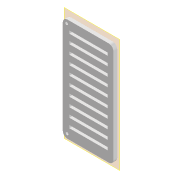
# Autodesk Inventor part: 00_Case_Powersupply_Galvo_lid
Saved by Autodesk Inventor 2022 (Build 260153000, 153)
## iProperties
Created: 2021-10-08
Part Number: 00_Case_Powersupply_Galvo_lid
Material: Generic
Document SubType Name: Modeling
Designer: wanghaoran
Density: 1 g/cm^3
Appearance: Default
Author: wanghaoran
Autodesk Inventor part; units mm, degrees
ref_plane "YZ Plane" through (0, 0, 0) normal (1, 0, 0) x (0, 1, 0)
ref_plane "XZ Plane" through (0, 0, 0) normal (0, 1, 0) x (-1, 0, 0)
ref_plane "XY Plane" through (0, 0, 0) normal (0, 0, 1) x (1, 0, 0)
ref_plane "Work Plane1" through (0, 0, 0) normal (0, 0, 1) x (1, 0, 0)
sketch "Sketch1" plane through (0, 0, 0) normal (0, 0, 1) x (1, 0, 0)
  circle A0 centre (-23, 51) radius 1.45 projected
  circle A1 centre (-22.4561, -50.4561) radius 1.45 projected
  arc A2 (-27, -50) -> (-22, -55) centre (-22, -50) ccw projected
  line L0 (-22, -55) -> (22, -55) projected
  arc A3 (22, -55) -> (27, -50) centre (22, -50) ccw projected
  line L1 (27, -50) -> (27, 50) projected
  arc A4 (27, 50) -> (22, 55) centre (22, 50) ccw projected
  line L2 (22, 55) -> (-22, 55) projected
  arc A5 (-22, 55) -> (-27, 50) centre (-22, 50) ccw projected
  line L3 (-27, 50) -> (-27, -50) projected
  line L4 (-22, 53) -> (22, 53) projected
  arc A6 (25, 50) -> (22, 53) centre (22, 50) ccw projected
  line L5 (25, 50) -> (25, -50) projected
  arc A7 (22, -53) -> (25, -50) centre (22, -50) ccw projected
  line L6 (22, -53) -> (-22, -53) projected
  arc A8 (-22, -53) -> (-25, -50) centre (-22.4561, -50.4561) ccw projected
  line L7 (-25, -50) -> (-25, 50) projected
  arc A9 (-25, 50) -> (-22, 53) centre (-23, 51) ccw projected
  point P0 (0, 0)
extrude "Extrusion1" add sketch "Sketch1" along normal blind 4 contours L3 A5 L2 A4 L1 A3 L0 A2 | L4 A6 L5 A7 L6 A8 L7 A9
sketch "Sketch2" plane through (0, 0, 0) normal (0, 0, -1) x (-1, 0, 0)
  line L0 (-25, 50) -> (-25, -50) projected
  line L1 (-25, 50) -> (-21, 50)
  line L2 (-21, 50) -> (-21, -50)
  line L3 (-21, -50) -> (-25, -50)
  line L4 (-25, -50) -> (-25, 50)
  line L5 (-21, 50) -> (-25, 50)
  line L6 (-25, 50) -> (-25, 51.5)
  line L7 (-25, 51.5) -> (-21, 51.5)
  line L8 (-21, 51.5) -> (-21, 50)
  line L9 (-21, -50) -> (-25, -50)
  line L10 (-25, -50) -> (-25, -51.5)
  line L11 (-25, -51.5) -> (-21, -51.5)
  line L12 (-21, -51.5) -> (-21, -50)
  point P0 (0, 0)
  dimension "d2" = 4
  dimension "d15" = 1.5
  dimension "d16" = 1.5
  constraints: 24 end point, 6 parallel, 3 horizontal, 3 perpendicular, 1 point on line
  measures "d2" distance of L2.end L3.end
  measures "d15" distance of L5.end L6.end
  measures "d16" distance of L10.end L9.end
extrude "Extrusion2" cut sketch "Sketch2" against normal blind 2
sketch "Sketch3" plane through (0, 0, 4) normal (0, 0, 1) x (1, 0, 0)
  line L0 (21, 50) -> (21, -50) projected
  line L1 (-20, 46) -> (21, 46)
  line L2 (21, 46) -> (21, 43)
  line L3 (21, 43) -> (-20, 43)
  line L4 (-20, 43) -> (-20, 46)
  line L5 (21, 33.3) -> (-20, 33.3)
  line L6 (-20, 36.3) -> (21, 36.3)
  line L7 (21, 36.3) -> (21, 33.3)
  line L8 (-20, 33.3) -> (-20, 36.3)
  line L9 (21, 23.6) -> (-20, 23.6)
  line L10 (-20, 26.6) -> (21, 26.6)
  line L11 (21, 26.6) -> (21, 23.6)
  line L12 (-20, 23.6) -> (-20, 26.6)
  line L13 (21, 13.9) -> (-20, 13.9)
  line L14 (-20, 16.9) -> (21, 16.9)
  line L15 (21, 16.9) -> (21, 13.9)
  line L16 (-20, 13.9) -> (-20, 16.9)
  line L17 (21, 4.2) -> (-20, 4.2)
  line L18 (-20, 7.2) -> (21, 7.2)
  line L19 (21, 7.2) -> (21, 4.2)
  line L20 (-20, 4.2) -> (-20, 7.2)
  line L21 (21, -5.5) -> (-20, -5.5)
  line L22 (-20, -2.5) -> (21, -2.5)
  line L23 (21, -2.5) -> (21, -5.5)
  line L24 (-20, -5.5) -> (-20, -2.5)
  line L25 (21, -15.2) -> (-20, -15.2)
  line L26 (-20, -12.2) -> (21, -12.2)
  line L27 (21, -12.2) -> (21, -15.2)
  line L28 (-20, -15.2) -> (-20, -12.2)
  line L29 (21, -24.9) -> (-20, -24.9)
  line L30 (-20, -21.9) -> (21, -21.9)
  line L31 (21, -21.9) -> (21, -24.9)
  line L32 (-20, -24.9) -> (-20, -21.9)
  line L33 (21, -34.6) -> (-20, -34.6)
  line L34 (-20, -31.6) -> (21, -31.6)
  line L35 (21, -31.6) -> (21, -34.6)
  line L36 (-20, -34.6) -> (-20, -31.6)
  line L37 (21, -44.3) -> (-20, -44.3)
  line L38 (-20, -41.3) -> (21, -41.3)
  line L39 (21, -41.3) -> (21, -44.3)
  line L40 (-20, -44.3) -> (-20, -41.3)
  line L41 (22, 55) -> (-22, 55) projected
  point P0 (0, 0)
  point P1 (21, -41.3)
  point P2 (21, -31.6)
  point P3 (21, -21.9)
  point P4 (21, -12.2)
  point P5 (21, -2.5)
  point P6 (21, 7.2)
  point P7 (21, 16.9)
  point P8 (21, 26.6)
  point P9 (21, 36.3)
  point P10 (21, 46)
  dimension "d5" = 3
  dimension "d8" = 9.7
  dimension "d17" = 9
  constraints: 80 end point, 36 vertical alignment, 20 parallel, 18 collinear, 1 horizontal, 1 perpendicular, 2 other
  measures "d5" distance of L1.end L2.end
  measures "d8" distance of L2.end L5.start
  measures "d17" distance between parallel lines of L41 L1
extrude "Extrusion3" cut sketch "Sketch3" against normal through all
body "Solid1"
